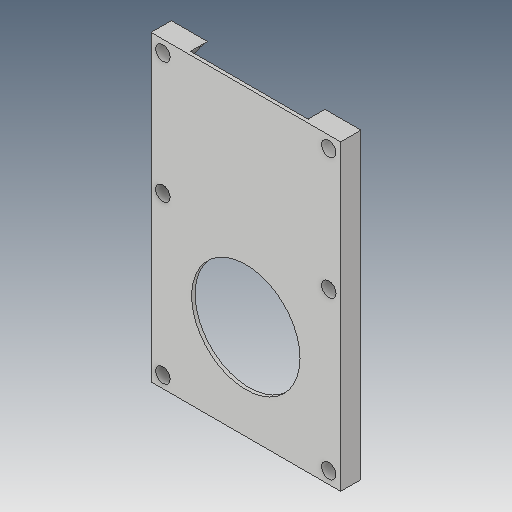
# Autodesk Inventor part: 200_Gearbox
Saved by Autodesk Inventor 2019 (Build 230136000, 136)
## iProperties
Created: 2019-07-08
Part Number: 200_Gearbox
Material: Generic
Document SubType Name: Modeling
Designer: diederichbenedict
Density: 1 g/cm^3
Appearance: Default
Author: diederichbenedict
Autodesk Inventor part; units mm, degrees
ref_plane "YZ Plane" through (0, 0, 0) normal (1, 0, 0) x (0, 1, 0)
ref_plane "XZ Plane" through (0, 0, 0) normal (0, 1, 0) x (-1, 0, 0)
ref_plane "XY Plane" through (0, 0, 0) normal (0, 0, 1) x (1, 0, 0)
sketch "Sketch1" plane through (0, 0, 0) normal (0, 0, 1) x (1, 0, 0)
  arc A0 (-7.3084, 9.5178) -> (7.3084, 9.5178) centre (0, 0) ccw
  arc A1 (8.2415, 16.5957) -> (9.4944, 19.0137) centre (0.0718, 22.3625) ccw construction
  line L0 (14, -14) -> (-14, -14)
  line L1 (-14, -14) -> (-14, 30.6843)
  line L2 (14, 30.6843) -> (14, -14)
  line L3 (7.3084, 12.4534) -> (7.3084, 9.5178)
  line L4 (-7.3084, 12.4534) -> (-7.3084, 9.5178)
  arc A2 (7.3084, 12.4534) -> (8.6716, 30.6843) centre (0, 22.1663) ccw
  arc A3 (-8.6716, 30.6843) -> (-7.3084, 12.4534) centre (0, 22.1663) ccw
  line L5 (-14, 30.6843) -> (-8.6716, 30.6843)
  line L6 (8.6716, 30.6843) -> (14, 30.6843)
  line L7 (-3.5, -3.5) -> (-3.5, 3.5) projected
  line L8 (-3.5, 3.5) -> (3.5, 3.5) projected
  line L9 (3.5, 3.5) -> (3.5, -3.5) projected
  line L10 (3.5, -3.5) -> (-3.5, -3.5) projected
  circle A4 centre (0, 0) radius 10 projected
  point P0 (0, 10)
  point P1 (-2.698, 9.6292)
  point P2 (-5.1958, 8.5442)
  point P3 (-7.3084, 6.8255)
  point P4 (-8.8789, 4.6007)
  point P5 (-9.7908, 2.0346)
  point P6 (-9.9767, -0.6824)
  point P7 (-9.4226, -3.3488)
  point P8 (-8.1697, -5.7668)
  point P9 (-6.3109, -7.7571)
  point P10 (-3.984, -9.1721)
  point P11 (-1.3617, -9.9069)
  point P12 (1.3617, -9.9069)
  point P13 (3.984, -9.1721)
  point P14 (6.3109, -7.7571)
  point P15 (8.1697, -5.7668)
  point P16 (9.4226, -3.3488)
  point P17 (9.9767, -0.6824)
  point P18 (9.7908, 2.0346)
  point P19 (8.8789, 4.6007)
  point P20 (7.3084, 6.8255)
  point P21 (5.1958, 8.5442)
  point P22 (2.698, 9.6292)
  point P23 (10.0485, 21.6801)
  dimension "d0" = 24
  dimension "d1" = 14
  dimension "d2" = 14
  dimension "d3" = 14
  constraints: 14 end point, 6 point on circle, 3 centre point, 3 parallel, 1 horizontal, 1 perpendicular, 2 other
  measures "d0" diameter of A0
  measures "d1" distance from line of point (0, 0) L2
  measures "d2" distance from line of L1 point (0, 0)
  measures "d3" distance from line of L0 point (0, 0)
extrude "Extrusion1" add sketch "Sketch1" against normal blind 2.5 contours A0 L3 A2 L6 L2 L0 L1 L5 A3 L4
sketch "Sketch2" plane through (0, 0, 0) normal (0, 0, 1) x (1, 0, 0)
  line L0 (14, -14) -> (-14, -14) projected
  line L1 (14, 30.6843) -> (14, -14) projected
  line L2 (8.6716, 30.6843) -> (14, 30.6843) projected
  arc A0 (7.3084, 12.4534) -> (8.6716, 30.6843) centre (0, 22.1663) ccw projected
  line L3 (7.3084, 9.5178) -> (7.3084, 12.4534) projected
  arc A1 (-7.3084, 9.5178) -> (7.3084, 9.5178) centre (0, 0) ccw projected
  line L4 (-7.3084, 12.4534) -> (-7.3084, 9.5178) projected
  arc A2 (-8.6716, 30.6843) -> (-7.3084, 12.4534) centre (0, 22.1663) ccw projected
  line L5 (-14, 30.6843) -> (-8.6716, 30.6843) projected
  line L6 (-14, -14) -> (-14, 30.6843) projected
  circle A3 centre (0, 0) radius 8
  line L7 (-14, 30.6843) -> (-8.6716, 30.6843) projected
  line L8 (8.6716, 30.6843) -> (-8.6716, 30.6843)
  dimension "d6" = 16
  constraints: 2 end point, 1 centre point, 1 coincident, 1 collinear
  measures "d6" diameter of A3
extrude "Extrusion2" add sketch "Sketch2" along normal blind 0.5
sketch "Sketch3" plane through (0, 0, -2.5) normal (0, 0, -1) x (-1, 0, 0)
  line L0 (-14, -14) -> (14, -14) projected
  line L1 (14, -14) -> (14, 30.6843) projected
  line L2 (14, 30.6843) -> (8.6716, 30.6843) projected
  arc A0 (7.3084, 12.4534) -> (8.6716, 30.6843) centre (0, 22.1663) ccw projected
  line L3 (7.3084, 12.4534) -> (7.3084, 9.5178) projected
  arc A1 (-7.3084, 9.5178) -> (7.3084, 9.5178) centre (0, 0) ccw projected
  line L4 (-7.3084, 9.5178) -> (-7.3084, 12.4534) projected
  arc A2 (-8.6716, 30.6843) -> (-7.3084, 12.4534) centre (0, 22.1663) ccw projected
  line L5 (-8.6716, 30.6843) -> (-14, 30.6843) projected
  line L6 (-14, 30.6843) -> (-14, -14) projected
  line L7 (12.2447, 28.929) -> (12.2447, -12.2447) construction
  line L8 (12.2447, -12.2447) -> (-12.2447, -12.2447) construction
  line L9 (-12.2447, -12.2447) -> (-12.2447, 28.929) construction
  line L10 (-12.2447, 28.929) -> (-12.1562, 28.929) construction
  arc A3 (-12.1562, 28.929) -> (-9.0637, 11.6137) centre (0, 22.1663) ccw construction
  line L11 (-9.0637, 11.6137) -> (-9.0637, 10.3469) construction
  arc A4 (-9.0637, 10.3469) -> (9.0637, 10.3469) centre (0, 0) ccw construction
  line L12 (9.0637, 10.3469) -> (9.0637, 11.6137) construction
  arc A5 (9.0637, 11.6137) -> (12.1562, 28.929) centre (0, 22.1663) ccw construction
  line L13 (12.1562, 28.929) -> (12.2447, 28.929) construction
  point P0 (12.2447, 10.9803)
  point P1 (-12.2447, 10.9803)
  constraints: 14 end point, 6 point on circle, 3 centre point, 2 point on line, 9 other
hole "Hole1" at (-12.2447, 10.9803, -2.5) at (12.2447, 10.9803, -2.5) at (-12.2447, 28.929, -2.5) at (-12.2447, -12.2447, -2.5) at (12.2447, -12.2447, -2.5) at (12.2447, 28.929, -2.5) direction (0, 0, 1) diameter 2.15 depth 16 tip angle 118
body "Solid1"
